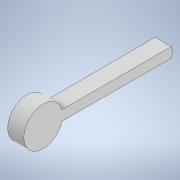
# Autodesk Inventor part: Pata2_v2
Saved by Autodesk Inventor 2021 (Build 250183000, 183)
## iProperties
Created: 2021-06-21
Part Number: Pata2_v2
Material: Genérico
Document SubType Name: Modeling
Designer: Juan
Density: 1 g/cm^3
Appearance: Valor por defecto
Author: Juan
Autodesk Inventor part; units mm, degrees
ref_plane "YZ Plane" through (0, 0, 0) normal (1, 0, 0) x (0, 1, 0)
ref_plane "XZ Plane" through (0, 0, 0) normal (0, 1, 0) x (-1, 0, 0)
ref_plane "XY Plane" through (0, 0, 0) normal (0, 0, 1) x (1, 0, 0)
sketch "Boceto1" plane through (0, 0, 0) normal (1, 0, 0) x (0, 1, 0)
  circle A0 centre (0, 0) radius 48
  dimension "d0" = 96
  constraints: 1 centre point, 1 coincident
  measures "d0" diameter of A0
extrude "Extrusión1" add sketch "Boceto1" along normal blind 40
sketch "Boceto2" plane through (40, 0, 0) normal (1, 0, 0) x (0, 0, -1)
  circle A0 centre (0, 0) radius 48 projected
  arc A1 (48, 0) -> (46.3644, 12.4233) centre (0, 0) ccw
  line L0 (0, 0) -> (46.3644, 12.4233) construction
  line L1 (0, 0) -> (48, 0) construction
  arc A2 (46.3644, -12.4233) -> (48, 0) centre (0, 0) ccw
  arc A3 (320.434, -0.0001) -> (317.7676, 12.4233) centre (290.159, -0.0001) ccw
  arc A4 (317.7677, -12.4233) -> (320.434, -0.0001) centre (290.159, -0.0001) ccw
  line L2 (46.3644, -12.4233) -> (317.7677, -12.4233)
  line L3 (317.7676, 12.4233) -> (46.3644, 12.4233)
  dimension "d3" = 15
  constraints: 11 point on circle, 8 end point, 4 centre point, 3 coincident, 2 concentric, 1 horizontal, 1 parallel
  measures "d3" angle of L1 L0
extrude "Extrusión2" add sketch "Boceto2" against normal blind 40 contours A0 L3 A3 A4 L2
